Rolling 60012RSSKF  12x28x8 mm (Autodesk Fusion 360 design; units mm, degrees)
Autodesk Fusion 360 part; units mm, degrees
sketch "Sketch1" plane through (0, 0, 0) normal (0, 0, 1) x (1, 0, 0)
  circle A0 centre (0, 0) radius 14
  circle A1 centre (0, 0) radius 6
  circle A2 centre (0, 0) radius 13
  circle A3 centre (0, 0) radius 8
  dimension "d1" = 28
  dimension "d2" = 12
  dimension "d5" = -1
  dimension "d6" = 2
  constraint coincident A0.centre A1.centre
  measures "d1" diameter of A0
  measures "d2" diameter of A1
extrude "Extrude2" add sketch "Sketch1" along normal blind 8 contours A0 makes body 1
fillet "Fillet1" radius 0.2 2 edges at (-13.0526, -5.0626, 8) (-12.1203, 4.701, 8) on bodies 1
fillet "Fillet1" radius 0.2 2 edges at (-13.0526, -5.0626, 0) (-12.1203, 4.701, 0) on bodies 1
extrude "Extrude3" add sketch "Sketch1" along normal blind 8 separate body contours A3 makes body 2
fillet "Fillet2" radius 0.2 2 edges at (-7.4586, -2.8929, 8) (-5.594, 2.1697, 8) on bodies 2
fillet "Fillet2" radius 0.2 2 edges at (-7.4586, -2.8929, 0) (-5.594, 2.1697, 0) on bodies 2
extrude "Extrude4" add sketch "Sketch1" along normal blind 8 separate body contours A2 makes body 3
fillet "Fillet3" radius 0.2 2 edges at (-12.1203, -4.701, 8) (-7.4586, 2.8929, 8) on bodies 3
fillet "Fillet3" radius 0.2 2 edges at (-12.1203, -4.701, 0) (-7.4586, 2.8929, 0) on bodies 3
combine "Combine1" operation add target body 1 tool bodies 2 3
